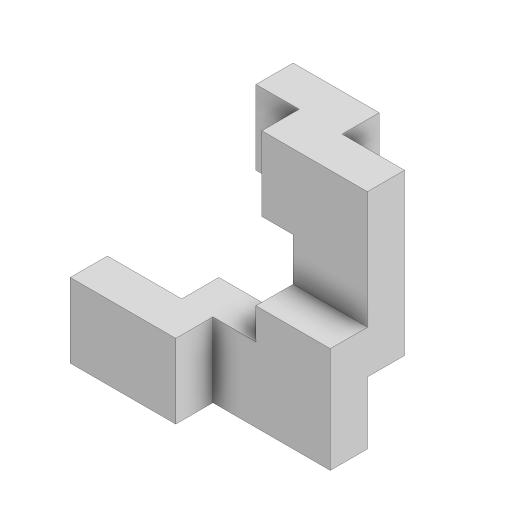
# Autodesk Inventor part: Template_ladder_2
Saved by Autodesk Inventor 2024 (Build 280153000, 153)
## iProperties
Created: 2023-03-18
Part Number: Template_ladder_2
Material: 一般
Document SubType Name: Modeling
Designer: USER
Density: 1 g/cm^3
Appearance: 預設
Author: USER
Autodesk Inventor part; units mm, degrees
ref_plane "YZ Plane" through (0, 0, 0) normal (1, 0, 0) x (0, 1, 0)
ref_plane "XZ Plane" through (0, 0, 0) normal (0, 1, 0) x (-1, 0, 0)
ref_plane "XY Plane" through (0, 0, 0) normal (0, 0, 1) x (1, 0, 0)
sketch "草圖15" plane through (0, 0, 0) normal (0, 0, 1) x (1, 0, 0)
  line L0 (5, -5) -> (-5, -5)
  line L1 (-5, -5) -> (-5, 5)
  line L2 (-5, 5) -> (5, 5)
  line L3 (5, 5) -> (5, -5)
  line L4 (5, -5) -> (-5, 5) construction
  line L5 (-5, -5) -> (5, 5) construction
  line L6 (15, -15) -> (-15, -15)
  line L7 (-15, -15) -> (-15, 15)
  line L8 (-15, 15) -> (15, 15)
  line L9 (15, 15) -> (15, -15)
  line L10 (15, -15) -> (-15, 15) construction
  line L11 (-15, -15) -> (15, 15) construction
  line L12 (-15, -15) -> (-0.8, -15)
  line L13 (-0.8, -15) -> (-0.8, -5)
  line L14 (-0.8, -5) -> (-15, -5)
  line L15 (-15, -5) -> (-15, -15)
  line L16 (15, -15) -> (-1.6, -15)
  line L17 (-1.6, -5) -> (15, -5)
  line L18 (15, -5) -> (15, -15)
  line L19 (15, -15) -> (5, -15)
  line L20 (5, -15) -> (5, -0.8)
  line L21 (5, -0.8) -> (15, -0.8)
  line L22 (15, -0.8) -> (15, -15)
  line L23 (15, 15) -> (5, 15)
  line L24 (5, 15) -> (5, -1.6)
  line L25 (15, -1.6) -> (15, 15)
  line L26 (15, 15) -> (0.8, 15)
  line L27 (0.8, 15) -> (0.8, 5)
  line L28 (0.8, 5) -> (15, 5)
  line L29 (15, 5) -> (15, 15)
  line L30 (-15, 15) -> (1.6, 15)
  line L31 (1.6, 5) -> (-15, 5)
  line L32 (-15, 5) -> (-15, 15)
  line L33 (-5, -5) -> (-15, -5)
  line L34 (-15, -5) -> (-15, -15)
  line L35 (-15, -15) -> (-5, -15)
  line L36 (-5, -15) -> (-5, -5)
  line L37 (-0.8, -15) -> (-6.6, -15)
  line L38 (-6.6, -15) -> (-6.6, -5)
  line L39 (-6.6, -5) -> (-0.8, -5)
  line L40 (-0.8, -5) -> (-0.8, -15)
  line L41 (5, -0.8) -> (15, -0.8)
  line L42 (15, -0.8) -> (15, -6.6)
  line L43 (15, -6.6) -> (5, -6.6)
  line L44 (5, -6.6) -> (5, -0.8)
  line L45 (0.8, 5) -> (6.6, 5)
  line L46 (6.6, 5) -> (6.6, 15)
  line L47 (6.6, 15) -> (0.8, 15)
  line L48 (0.8, 15) -> (0.8, 5)
  line L49 (0.8, 5) -> (-5, 5)
  line L50 (-5, 5) -> (-5, 15)
  line L51 (-5, 15) -> (0.8, 15)
  line L52 (0.8, 15) -> (0.8, 5)
  point P0 (0, 0)
  point P1 (0, 0)
  point P2 (-15, -5)
  point P3 (15, -0.8)
  point P4 (5, -15)
  point P5 (0.8, 15)
  point P6 (-15, 5)
  point P7 (-5, 5)
  point P8 (15, -5)
  point P9 (-5, -15)
  point P10 (5, 5)
  point P11 (5, 15)
  point P12 (0.8, 15)
  point P13 (-6.6, -5)
  point P14 (-6.6, -15)
  point P15 (5, -6.6)
  point P16 (15, -6.6)
  point P17 (-5, 5)
  point P18 (5, 5)
  point P19 (6.6, 5)
  point P20 (6.6, 15)
  dimension "d38" = 10
  dimension "d39" = 10
  dimension "d40" = 0.8
  dimension "d42" = 0.8
  dimension "d48" = 0.8
  dimension "d54" = 0
  dimension "d55" = 5.8
  dimension "d56" = 5.8
  dimension "d57" = 5.8
  dimension "d58" = 10
  constraints: 106 end point, 23 parallel, 13 horizontal, 13 perpendicular, 11 point on line, 4 midpoint, 1 coincident
  measures "d38" distance of L1.end L2.end
  measures "d39" distance between parallel lines of L8 L2
  measures "d40" distance from line of point (0, 0) L13
  measures "d42" distance from line of point (0, 0) L21
  measures "d48" distance from line of point (0, 0) L27
  measures "d54" distance between parallel lines of L7 L32
  measures "d55" distance between parallel lines of L38 L13
  measures "d56" distance between parallel lines of L41 L43
  measures "d57" distance between parallel lines of L27 L46
  measures "d58" distance between parallel lines of L50 L24
extrude "擠出10" add sketch "草圖15" against normal blind 5 contours L13 L6 L36 L0 | L36 L6 L38 L14 | L38 L6 L7 L14
extrude "擠出11" add sketch "草圖15" against normal blind 5 from surface at -5 contours L20 L6 L13 L0 | L3 L21 L9 L17 | L17 L9 L43 L20 | L13 L6 L36 L0 | L43 L9 L6 L20
extrude "擠出12" add sketch "草圖15" against normal blind 5 from surface at -10 contours L3 L21 L9 L17 | L17 L9 L43 L20 | L3 L28 L9 L21 | L2 L27 L8 L24 | L24 L8 L46 L28 | L46 L8 L9 L28
extrude "擠出13" add sketch "草圖15" against normal blind 5 from surface at -15 contours L2 L27 L8 L24 | L24 L8 L46 L28 | L50 L8 L27 L2
equation "\"d39\" = width"
equation "\"d40\" = gap"
equation "\"d42\" = gap"
equation "\"d48\" = gap"
equation "\"d55\" = stack"
equation "\"d56\" = stack"
equation "\"d57\" = stack"
equation "\"d44\" = height"
equation "\"d46\" = height"
equation "\"d50\" = height"
equation "\"d52\" = height"
equation "\"width\" = 10"
equation "\"height\" = 5"
equation "\"gap\" = 0.8"
equation "\"stack\" = 5.8"
